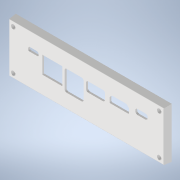
# Autodesk Inventor part: A-03
Saved by Autodesk Inventor 2022.2 (Build 262287000, 287)
## iProperties
Created: 2021-11-25
Part Number: A-03
Material: Generic
Document SubType Name: Modeling
Designer: kfcs7
Density: 1 g/cm^3
Appearance: Default
Author: kfcs7
Autodesk Inventor part; units mm, degrees
ref_plane "YZ Plane" through (0, 0, 0) normal (1, 0, 0) x (0, 1, 0)
ref_plane "XZ Plane" through (0, 0, 0) normal (0, 1, 0) x (-1, 0, 0)
ref_plane "XY Plane" through (0, 0, 0) normal (0, 0, 1) x (1, 0, 0)
sketch "Sketch1" plane through (0, 0, 0) normal (0, 0, 1) x (1, 0, 0)
  circle A0 centre (4, 4) radius 2.25 construction
  line L0 (119, 20) -> (119, 10.0711) construction
  line L1 (119, 10.0711) -> (113.9289, 5) construction
  line L2 (113.9289, 5) -> (10.0711, 5) construction
  line L3 (10.0711, 5) -> (5, 10.0711) construction
  line L4 (5, 10.0711) -> (5, 20) construction
  line L5 (0, 20) -> (5, 20) construction
  line L6 (0, 0) -> (0, 20) construction
  line L7 (124, 0) -> (0, 0) construction
  line L8 (124, 0) -> (124, 20) construction
  line L9 (119, 20) -> (124, 20) construction
  circle A1 centre (120, 4) radius 2.25 construction
  circle A2 centre (120, 36) radius 2.25 construction
  line L10 (119, 29.9289) -> (119, 20) construction
  line L11 (124, 20) -> (119, 20) construction
  line L12 (124, 40) -> (124, 20) construction
  line L13 (0, 40) -> (124, 40) construction
  line L14 (0, 20) -> (0, 40) construction
  line L15 (5, 20) -> (0, 20) construction
  line L16 (5, 20) -> (5, 29.9289) construction
  line L17 (5, 29.9289) -> (10.0711, 35) construction
  line L18 (10.0711, 35) -> (113.9289, 35) construction
  line L19 (113.9289, 35) -> (119, 29.9289) construction
  circle A3 centre (4, 36) radius 2.25 construction
  line L20 (124, 0) -> (0, 0)
  line L21 (0, 0) -> (0, 40)
  line L22 (0, 40) -> (124, 40)
  line L23 (124, 40) -> (124, 0)
  constraints: 8 end point, 2 parallel, 1 horizontal, 1 perpendicular
extrude "Extrusion1" add sketch "Sketch1" along normal blind 6 draft -5
sketch "Sketch2" plane through (0, 0, 6) normal (0, 0, 1) x (1, 0, 0)
  arc A0 (94.899, 22.2237) -> (95.649, 22.9616) centre (94.899, 22.9738) ccw construction
  line L0 (95.649, 25.4127) -> (95.649, 22.9616) construction
  arc A1 (95.649, 25.4127) -> (95.155, 26.0813) centre (94.949, 25.4122) ccw construction
  line L1 (94.6627, 26.2328) -> (95.155, 26.0812) construction
  ellipse E0 centre (94.838, 26.8064) end of major axis (95.2338, 26.3557) minor radius 0.5998 (94.3875, 26.4105) -> (94.6627, 26.2328) ccw construction
  line L2 (93.563, 27.3474) -> (94.3875, 26.4104) construction
  arc A2 (93.563, 27.3474) -> (93.0394, 27.5839) centre (93.0384, 26.8838) ccw construction
  line L3 (93.0394, 27.5839) -> (87.764, 27.5838) construction
  line L4 (93.0394, 27.3839) -> (87.764, 27.3838) construction
  arc A3 (93.4133, 27.2149) -> (93.0394, 27.3839) centre (93.0385, 26.884) ccw construction
  line L5 (93.4132, 27.2148) -> (94.2371, 26.2786) construction
  arc A4 (94.2371, 26.2786) -> (94.6032, 26.0418) centre (94.838, 26.8064) ccw construction
  line L6 (94.6032, 26.0418) -> (95.0963, 25.8901) construction
  arc A5 (95.449, 25.4123) -> (95.0963, 25.8901) centre (94.9491, 25.4123) ccw construction
  line L7 (95.449, 25.4123) -> (95.449, 22.9838) construction
  arc A6 (94.899, 22.4338) -> (95.449, 22.9838) centre (94.899, 22.9838) ccw construction
  line L8 (94.899, 22.4338) -> (81.599, 22.4338) construction
  arc A7 (81.049, 22.9838) -> (81.599, 22.4338) centre (81.599, 22.9838) ccw construction
  line L9 (81.049, 25.4124) -> (81.049, 22.9838) construction
  arc A8 (81.4019, 25.8901) -> (81.049, 25.4124) centre (81.549, 25.4123) ccw construction
  line L10 (81.4019, 25.8901) -> (81.8946, 26.0417) construction
  arc A9 (81.8946, 26.0417) -> (82.2607, 26.2783) centre (81.66, 26.8064) ccw construction
  line L11 (82.2608, 26.2783) -> (83.0849, 27.2149) construction
  arc A10 (83.4586, 27.3839) -> (83.0849, 27.215) centre (83.4596, 26.884) ccw construction
  line L12 (83.4586, 27.3839) -> (87.734, 27.3838) construction
  line L13 (83.4592, 27.5839) -> (87.734, 27.5838) construction
  arc A11 (83.4591, 27.5839) -> (82.9343, 27.3465) centre (83.4596, 26.8838) ccw construction
  line L14 (82.1104, 26.4103) -> (82.9343, 27.3465) construction
  arc A12 (81.8359, 26.2329) -> (82.1104, 26.4103) centre (81.6598, 26.8063) ccw construction
  line L15 (81.8359, 26.2329) -> (81.3425, 26.0811) construction
  arc A13 (81.3425, 26.0811) -> (80.849, 25.4126) centre (81.549, 25.4122) ccw construction
  line L16 (80.849, 22.9616) -> (80.849, 25.4126) construction
  arc A14 (80.849, 22.9616) -> (81.599, 22.2237) centre (81.599, 22.9738) ccw construction
  line L17 (94.899, 22.2237) -> (81.599, 22.2237) construction
  arc A15 (110.415, 27.0138) -> (109.085, 28.3438) centre (109.085, 27.0138) ccw construction
  line L18 (105.945, 28.3438) -> (109.085, 28.3438) construction
  line L19 (105.945, 28.1938) -> (109.085, 28.1938) construction
  arc A16 (110.265, 27.0138) -> (109.085, 28.1938) centre (109.085, 27.0138) ccw construction
  line L20 (110.265, 27.0138) -> (110.265, 26.5138) construction
  arc A17 (109.085, 25.3338) -> (110.265, 26.5138) centre (109.085, 26.5138) ccw construction
  line L21 (109.085, 25.3338) -> (102.805, 25.3338) construction
  arc A18 (101.625, 26.5138) -> (102.805, 25.3338) centre (102.805, 26.5138) ccw construction
  line L22 (101.625, 26.5138) -> (101.625, 27.0138) construction
  arc A19 (102.805, 28.1938) -> (101.625, 27.0138) centre (102.805, 27.0138) ccw construction
  line L23 (102.805, 28.1938) -> (105.895, 28.1938) construction
  line L24 (102.805, 28.3438) -> (105.895, 28.3438) construction
  arc A20 (102.805, 28.3438) -> (101.475, 27.0138) centre (102.805, 27.0138) ccw construction
  line L25 (101.475, 27.0138) -> (101.475, 26.5138) construction
  arc A21 (101.475, 26.5138) -> (102.805, 25.1838) centre (102.805, 26.5138) ccw construction
  line L26 (109.085, 25.1838) -> (102.805, 25.1838) construction
  arc A22 (109.085, 25.1838) -> (110.415, 26.5138) centre (109.085, 26.5138) ccw construction
  line L27 (110.415, 27.0138) -> (110.415, 26.5138) construction
  line L28 (42.15, 27.38) -> (37.55, 27.38) construction
  line L29 (42.15, 27.38) -> (42.15, 25.03) construction
  line L30 (42.15, 25.03) -> (41.5, 25.03) construction
  line L31 (41.5, 25.03) -> (41.5, 23.13) construction
  line L32 (41.5, 23.13) -> (41.7, 23.13) construction
  arc A23 (41.7, 22.73) -> (41.7, 23.13) centre (41.7, 22.93) ccw construction
  line L33 (41.7, 22.73) -> (41.5, 22.73) construction
  line L34 (41.5, 22.73) -> (41.5, 20.73) construction
  line L35 (41.5, 20.73) -> (41.7, 20.73) construction
  arc A24 (41.7, 20.33) -> (41.7, 20.73) centre (41.7, 20.53) ccw construction
  line L36 (41.7, 20.33) -> (41.5, 20.33) construction
  line L37 (41.5, 17.06) -> (41.5, 20.33) construction
  line L38 (41.5, 17.06) -> (28.6, 17.06) construction
  line L39 (28.6, 17.06) -> (28.6, 20.33) construction
  line L40 (28.6, 20.33) -> (28.4, 20.33) construction
  arc A25 (28.4, 20.73) -> (28.4, 20.33) centre (28.4, 20.53) ccw construction
  line L41 (28.4, 20.73) -> (28.6, 20.73) construction
  line L42 (28.6, 20.73) -> (28.6, 22.73) construction
  line L43 (28.6, 22.73) -> (28.4, 22.73) construction
  arc A26 (28.4, 23.13) -> (28.4, 22.73) centre (28.4, 22.93) ccw construction
  line L44 (28.4, 23.13) -> (28.6, 23.13) construction
  line L45 (28.6, 25.03) -> (28.6, 23.13) construction
  line L46 (28.6, 25.03) -> (27.95, 25.03) construction
  line L47 (27.95, 25.03) -> (27.95, 27.38) construction
  line L48 (32.55, 27.38) -> (27.95, 27.38) construction
  line L49 (32.55, 27.83) -> (28.05, 27.83) construction
  line L50 (27.5, 27.83) -> (28.05, 27.83) construction
  line L51 (27.5, 27.83) -> (27.5, 15.13) construction
  line L52 (27.5, 15.13) -> (42.6, 15.13) construction
  line L53 (42.6, 15.13) -> (42.6001, 27.83) construction
  line L54 (42.05, 27.83) -> (42.6001, 27.83) construction
  line L55 (42.05, 27.83) -> (37.55, 27.8299) construction
  arc A27 (75.95, 26.59) -> (75.35, 27.19) centre (75.35, 26.59) ccw construction
  arc A28 (75.35, 21.47) -> (75.95, 22.07) centre (75.35, 22.07) ccw construction
  arc A29 (62.85, 22.07) -> (63.45, 21.47) centre (63.45, 22.07) ccw construction
  arc A30 (63.45, 27.19) -> (62.85, 26.59) centre (63.45, 26.59) ccw construction
  arc A31 (16.3, 26.3538) -> (16.7, 25.9538) centre (16.7, 26.3538) ccw construction
  arc A32 (23.3, 25.9538) -> (23.7, 26.3538) centre (23.3, 26.3538) ccw construction
  line L56 (22.9207, 28.1866) -> (23.5829, 27.5245) construction
  line L57 (17.0793, 28.1866) -> (16.4172, 27.5245) construction
  arc A33 (46.35, 27.26) -> (45.85, 26.76) centre (46.35, 26.76) ccw construction
  arc A34 (58.95, 26.76) -> (58.45, 27.26) centre (58.45, 26.76) ccw construction
  arc A35 (58.45, 12.88) -> (58.95, 13.38) centre (58.45, 13.38) ccw construction
  arc A36 (45.85, 13.38) -> (46.35, 12.88) centre (46.35, 13.38) ccw construction
  line L58 (75.35, 21.47) -> (63.45, 21.47) construction
  line L59 (62.85, 22.07) -> (62.85, 26.59) construction
  line L60 (63.45, 27.19) -> (75.35, 27.19) construction
  line L61 (75.95, 26.59) -> (75.95, 22.07) construction
  line L62 (58.95, 13.38) -> (58.95, 26.76) construction
  line L63 (45.85, 26.76) -> (45.85, 13.38) construction
  line L64 (46.35, 12.88) -> (58.45, 12.88) construction
  line L65 (58.45, 27.26) -> (46.35, 27.26) construction
  line L66 (37.55, 27.8299) -> (32.55, 27.83) construction
  line L67 (22.9207, 28.1866) -> (17.0793, 28.1866) construction
  line L68 (16.4172, 27.5245) -> (16.3, 26.3538) construction
  line L69 (16.7, 25.9538) -> (23.3, 25.9538) construction
  line L70 (23.7, 26.3538) -> (23.5829, 27.5245) construction
  line L71 (105.945, 28.3438) -> (105.895, 28.3438) construction
  line L72 (105.945, 28.1938) -> (105.895, 28.1938) construction
  arc A37 (109.085, 24.6838) -> (110.915, 26.5138) centre (109.085, 26.5138) ccw
  line L73 (109.085, 24.6838) -> (102.805, 24.6838)
  arc A38 (100.975, 26.5138) -> (102.805, 24.6838) centre (102.805, 26.5138) ccw
  line L74 (100.975, 26.5138) -> (100.975, 27.0138)
  arc A39 (102.805, 28.8438) -> (100.975, 27.0138) centre (102.805, 27.0138) ccw
  line L75 (102.805, 28.8438) -> (105.895, 28.8438)
  line L76 (105.895, 28.8438) -> (105.945, 28.8438)
  line L77 (105.945, 28.8438) -> (109.085, 28.8438)
  arc A40 (110.915, 27.0138) -> (109.085, 28.8438) centre (109.085, 27.0138) ccw
  line L78 (110.915, 27.0138) -> (110.915, 26.5138)
  line L79 (87.764, 27.5838) -> (87.734, 27.5838) construction
  line L80 (87.764, 27.3838) -> (87.734, 27.3838) construction
  line L81 (88.249, 22.4338) -> (88.2489, 27.3838) construction
  line L82 (95.999, 21.9088) -> (80.499, 21.9088)
  line L83 (80.499, 21.9088) -> (80.499, 27.9088)
  line L84 (80.499, 27.9088) -> (95.999, 27.9088)
  line L85 (95.999, 27.9088) -> (95.999, 21.9088)
  line L86 (95.999, 21.9088) -> (80.499, 27.9088) construction
  line L87 (80.499, 21.9088) -> (95.999, 27.9088) construction
  arc A41 (61.85, 22.07) -> (63.45, 20.47) centre (63.45, 22.07) ccw
  line L88 (61.85, 22.07) -> (61.85, 26.59)
  arc A42 (63.45, 28.19) -> (61.85, 26.59) centre (63.45, 26.59) ccw
  line L89 (63.45, 28.19) -> (75.35, 28.19)
  arc A43 (76.95, 26.59) -> (75.35, 28.19) centre (75.35, 26.59) ccw
  line L90 (76.95, 26.59) -> (76.95, 22.07)
  arc A44 (75.35, 20.47) -> (76.95, 22.07) centre (75.35, 22.07) ccw
  line L91 (75.35, 20.47) -> (63.45, 20.47)
  arc A45 (59.95, 26.76) -> (58.45, 28.26) centre (58.45, 26.76) ccw
  line L92 (58.45, 28.26) -> (46.35, 28.26)
  arc A46 (46.35, 28.26) -> (44.85, 26.76) centre (46.35, 26.76) ccw
  line L93 (44.85, 26.76) -> (44.85, 13.38)
  arc A47 (44.85, 13.38) -> (46.35, 11.88) centre (46.35, 13.38) ccw
  line L94 (46.35, 11.88) -> (58.45, 11.88)
  arc A48 (58.45, 11.88) -> (59.95, 13.38) centre (58.45, 13.38) ccw
  line L95 (59.95, 13.38) -> (59.95, 26.76)
  line L96 (42.6, 15.13) -> (27.5, 15.13) construction
  line L97 (27.5, 15.13) -> (27.5, 27.83)
  line L98 (27.5, 27.83) -> (42.6, 27.83) construction
  line L99 (42.6, 27.83) -> (42.6, 15.13) construction
  line L100 (27, 14.63) -> (43.1, 14.63)
  line L101 (43.1, 14.63) -> (43.1, 28.33)
  line L102 (43.1, 28.33) -> (27, 28.33)
  line L103 (27, 28.33) -> (27, 14.63)
  line L104 (16.8722, 28.6866) -> (15.9374, 27.7519)
  line L105 (15.9374, 27.7519) -> (15.8005, 26.3837)
  arc A49 (15.8005, 26.3837) -> (16.7, 25.4538) centre (16.7, 26.3538) ccw
  line L106 (16.7, 25.4538) -> (23.3, 25.4538)
  arc A50 (23.3, 25.4538) -> (24.1995, 26.3837) centre (23.3, 26.3538) ccw
  line L107 (24.1995, 26.3837) -> (24.0626, 27.7519)
  line L108 (24.0626, 27.7519) -> (23.1278, 28.6866)
  line L109 (23.1278, 28.6866) -> (16.8722, 28.6866)
  point P0 (0, 0)
  point P1 (88.249, 24.9088)
  dimension "d2" = 0.5
  dimension "d3" = 15.5
  dimension "d4" = 6
  dimension "d5" = 1
  dimension "d6" = 1
  dimension "d7" = 0.5
  dimension "d8" = 0.5
  constraints: 104 end point, 28 point on circle, 14 centre point, 13 parallel, 12 perpendicular, 4 horizontal, 4 midpoint, 3 collinear, 1 point on line, 1 tangent, 34 other
  measures "d2" radial gap between concentric circles of A22 A37
  measures "d3" distance of L83.end L84.end
  measures "d4" distance of L82.end L83.end
  measures "d5" distance between parallel lines of L58 L91
  measures "d6" distance between parallel lines of L62 L95
  measures "d7" distance between parallel lines of L96 L100
  measures "d8" distance between parallel lines of L67 L109
extrude "Extrusion2" cut sketch "Sketch2" against normal through all
chamfer "Chamfer1" distance 2 angle 45 2 edges at (95.999, 27.9088, 3) (80.499, 27.9088, 3)
chamfer "Chamfer2" distance 0.5 angle 45 2 edges at (95.999, 21.9088, 3) (80.499, 21.9088, 3)
sketch "Sketch4" plane through (0, 0, 0) normal (0, 0, -1) x (-1, 0, 0)
  arc A0 (-16.7, 25.4538) -> (-15.8005, 26.3837) centre (-16.7, 26.3538) ccw construction
  line L0 (-16.7, 25.4538) -> (-23.3, 25.4538) construction
  arc A1 (-24.1995, 26.3837) -> (-23.3, 25.4538) centre (-23.3, 26.3538) ccw construction
  line L1 (-24.1995, 26.3837) -> (-24.0626, 27.7519) construction
  line L2 (-24.0626, 27.7519) -> (-23.1278, 28.6866) construction
  line L3 (-23.1278, 28.6866) -> (-16.8722, 28.6866) construction
  line L4 (-16.8722, 28.6866) -> (-15.9374, 27.7519) construction
  line L5 (-15.9374, 27.7519) -> (-15.8005, 26.3837) construction
  arc A2 (-63.45, 20.47) -> (-61.85, 22.07) centre (-63.45, 22.07) ccw construction
  line L6 (-63.45, 20.47) -> (-75.35, 20.47) construction
  arc A3 (-76.95, 22.07) -> (-75.35, 20.47) centre (-75.35, 22.07) ccw construction
  line L7 (-76.95, 22.07) -> (-76.95, 26.59) construction
  arc A4 (-75.35, 28.19) -> (-76.95, 26.59) centre (-75.35, 26.59) ccw construction
  line L8 (-75.35, 28.19) -> (-63.45, 28.19) construction
  arc A5 (-61.85, 26.59) -> (-63.45, 28.19) centre (-63.45, 26.59) ccw construction
  line L9 (-61.85, 26.59) -> (-61.85, 22.07) construction
  arc A6 (-44.85, 26.76) -> (-46.35, 28.26) centre (-46.35, 26.76) ccw construction
  line L10 (-44.85, 26.76) -> (-44.85, 13.38) construction
  arc A7 (-46.35, 11.88) -> (-44.85, 13.38) centre (-46.35, 13.38) ccw construction
  line L11 (-46.35, 11.88) -> (-58.45, 11.88) construction
  arc A8 (-59.95, 13.38) -> (-58.45, 11.88) centre (-58.45, 13.38) ccw construction
  line L12 (-59.95, 13.38) -> (-59.95, 26.76) construction
  arc A9 (-58.45, 28.26) -> (-59.95, 26.76) centre (-58.45, 26.76) ccw construction
  line L13 (-58.45, 28.26) -> (-46.35, 28.26) construction
  arc A10 (-110.915, 26.5138) -> (-109.085, 24.6838) centre (-109.085, 26.5138) ccw construction
  line L14 (-110.915, 26.5138) -> (-110.915, 27.0138) construction
  arc A11 (-109.085, 28.8438) -> (-110.915, 27.0138) centre (-109.085, 27.0138) ccw construction
  line L15 (-109.085, 28.8438) -> (-102.805, 28.8438) construction
  arc A12 (-100.975, 27.0138) -> (-102.805, 28.8438) centre (-102.805, 27.0138) ccw construction
  line L16 (-100.975, 27.0138) -> (-100.975, 26.5138) construction
  arc A13 (-102.805, 24.6838) -> (-100.975, 26.5138) centre (-102.805, 26.5138) ccw construction
  line L17 (-102.805, 24.6838) -> (-109.085, 24.6838) construction
  line L18 (-80.499, 25.9088) -> (-80.499, 22.4088) construction
  line L19 (-80.999, 21.9088) -> (-80.499, 22.4088) construction
  line L20 (-80.999, 21.9088) -> (-95.499, 21.9088) construction
  line L21 (-95.999, 22.4088) -> (-95.499, 21.9088) construction
  line L22 (-95.999, 22.4088) -> (-95.999, 25.9088) construction
  line L23 (-93.999, 27.9088) -> (-95.999, 25.9088) construction
  line L24 (-93.999, 27.9088) -> (-82.499, 27.9088) construction
  line L25 (-80.499, 25.9088) -> (-82.499, 27.9088) construction
  line L26 (-43.1, 28.33) -> (-27, 28.33) construction
  line L27 (-27, 28.33) -> (-27, 14.63) construction
  line L28 (-27, 14.63) -> (-43.1, 14.63) construction
  line L29 (-43.1, 14.63) -> (-43.1, 28.33) construction
  line L30 (-124, 40) -> (0, 40) construction
  line L31 (-124, 0) -> (-124, 40) construction
  line L32 (0, 0) -> (-124, 0) construction
  line L33 (0, 40) -> (0, 0) construction
  circle A14 centre (-120, 4) radius 2.25 construction
  line L34 (-119, 10.0711) -> (-119, 20) projected
  line L35 (-124, 20) -> (-119, 20) construction
  line L36 (-124, 0) -> (-124, 20) construction
  line L37 (0, 0) -> (-124, 0) construction
  line L38 (0, 20) -> (0, 0) construction
  line L39 (-5, 20) -> (0, 20) construction
  line L40 (-5, 20) -> (-5, 10.0711) projected
  line L41 (-5, 10.0711) -> (-10.0711, 5) projected
  line L42 (-10.0711, 5) -> (-113.9289, 5) projected
  line L43 (-113.9289, 5) -> (-119, 10.0711) projected
  circle A15 centre (-4, 4) radius 2.25 construction
  circle A16 centre (-4, 36) radius 2.25 construction
  line L44 (-119, 20) -> (-119, 29.9289) projected
  line L45 (-119, 29.9289) -> (-113.9289, 35) projected
  line L46 (-113.9289, 35) -> (-10.0711, 35) projected
  line L47 (-10.0711, 35) -> (-5, 29.9289) projected
  line L48 (-5, 29.9289) -> (-5, 20) projected
  line L49 (0, 20) -> (-5, 20) construction
  line L50 (0, 40) -> (0, 20) construction
  line L51 (-124, 40) -> (0, 40) construction
  line L52 (-124, 40) -> (-124, 20) construction
  line L53 (-119, 20) -> (-124, 20) construction
  circle A17 centre (-120, 36) radius 2.25 construction
extrude "Extrusion4" cut sketch "Sketch4" against normal blind 4.5 draft -25
sketch "Sketch5" plane through (0, 0, 6) normal (0, 0, 1) x (1, 0, 0)
  circle A0 centre (120, 4) radius 1.7718 projected
  circle A1 centre (120, 36) radius 1.7718 projected
  circle A2 centre (4, 36) radius 1.7718 projected
  circle A3 centre (4, 4) radius 1.7718 projected
  point P0 (0, 0)
extrude "Extrusion5" cut sketch "Sketch5" against normal through all
fillet "Fillet1" radius 0.5 4 edges at (62, 0.5249, 6) (123.4751, 20, 6) (62, 39.4751, 6) (0.5249, 20, 6)
body "Solid1"
